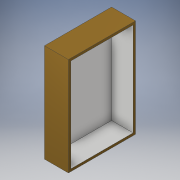
# Autodesk Inventor part: IPRO Carlos Case
Saved by Autodesk Inventor 2018 (Build 220112000, 112)
## iProperties
Created: 2019-03-20
Part Number: IPRO Carlos Case
Material: Generic
Document SubType Name: Modeling
Designer: Music X
Density: 1 g/cm^3
Appearance: Default
Author: Music X
Autodesk Inventor part; units mm, degrees
ref_plane "YZ Plane" through (0, 0, 0) normal (1, 0, 0) x (0, 1, 0)
ref_plane "XZ Plane" through (0, 0, 0) normal (0, 1, 0) x (-1, 0, 0)
ref_plane "XY Plane" through (0, 0, 0) normal (0, 0, 1) x (1, 0, 0)
sketch "Sketch1" plane through (0, 0, 0) normal (1, 0, 0) x (0, 1, 0)
  line L0 (0, 0) -> (82, 0)
  line L1 (82, 0) -> (82, -56)
  line L2 (82, -56) -> (0, -56)
  line L3 (0, -56) -> (0, 0)
  dimension "d0" = 82
  dimension "d1" = 56
  constraints: 8 end point, 2 parallel, 1 horizontal, 1 perpendicular
  measures "d0" distance of L1.end L2.end
  measures "d1" distance of L0.end L1.end
extrude "Extrusion1" add sketch "Sketch1" along normal blind 20
shell "Shell1" thickness 2 removed faces 1 at (20, 27.3333, -18.6667)
body "Solid1"
